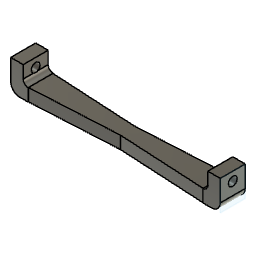
refuerzo estructura brazo elevador (Autodesk Fusion 360 design; units mm, degrees)
Autodesk Fusion 360 part; units mm, degrees
sketch "Sketch1" plane through (0, 0, 0) normal (0, 0, 1) x (1, 0, 0)
  line L0 (0, 0) -> (84, 0)
  line L1 (84, 0) -> (84, 10)
  line L2 (84, 10) -> (0, 10)
  line L3 (0, 10) -> (0, 0)
  dimension "d1" = 84
  dimension "d2" = 10
  constraint horizontal L0
  constraint vertical L1
  constraint horizontal L2
  constraint vertical L3
  constraint coincident L0.start L3.end
  measures "d1" distance of L0.start L0.end
  measures "d2" distance of L0.start L2.end
extrude "Extrude1" add sketch "Sketch1" along normal blind 12
sketch "Sketch2" plane through (0, 0, 0) normal (0, -1, 0) x (1, 0, 0)
  line L0 (0, 0) -> (84, 0)
  line L1 (84, 0) -> (84, 12)
  line L2 (84, 12) -> (0, 12)
  line L3 (0, 12) -> (0, 0)
sketch "Sketch3" plane through (0, 0, 0) normal (0, -1, 0) x (1, 0, 0)
  line L0 (0, 12) -> (5, 12)
  line L1 (5, 12) -> (5, 5)
  line L2 (5, 5) -> (79, 5)
  line L3 (5, 12) -> (6.9617, 12)
  line L4 (6.9617, 12) -> (80, 12)
  line L5 (84, 12) -> (79, 12)
  line L6 (79, 12) -> (79, 5)
  dimension "d5" = 5
  constraint horizontal L0
  constraint perpendicular L0 L1
  constraint perpendicular L1 L2
  constraint perpendicular L1 L3
  constraint parallel L4 L5
  constraint coincident L2 L6.end
  constraint perpendicular L2 L6
  measures "d5" distance of L5.start L5.end
extrude "Extrude2" cut sketch "Sketch3" against normal blind 50
sketch "Sketch4" plane through (84, 0, 0) normal (1, 0, 0) x (0, 1, 0)
  line L0 (0, 0) -> (10, 0)
  line L1 (10, 0) -> (10, 12)
  line L2 (10, 12) -> (0, 12)
  line L3 (0, 12) -> (0, 0)
sketch "Sketch5" plane through (79, 0, 0) normal (-1, 0, 0) x (0, -1, 0)
  line L0 (-10, 12) -> (-10, 5)
  line L1 (-10, 5) -> (0, 5)
  line L2 (0, 5) -> (0, 12)
  line L3 (0, 12) -> (-10, 12)
  circle A0 centre (-5, 8.5) radius 1.75
  dimension "d8" = 3.5
  measures "d8" diameter of A0
extrude "Extrude3" cut sketch "Sketch5" along normal blind 162 and the other way blind 9 contours A0
fillet "Fillet1" radius 3.5 2 edges at (84, 5, 0) (0, 5, 0)
fillet "Fillet2" radius 2 2 edges at (5, 5, 5) (79, 5, 5)
sketch "Sketch6" plane through (0, 0, 5) normal (0, 0, 1) x (-1, 0, 0)
  line L0 (-77, 0) -> (-77, -10)
  line L1 (-77, -10) -> (-7, -10)
  line L2 (-7, -10) -> (-7, 0)
  line L3 (-7, 0) -> (-77, 0)
  line L4 (-42, 0) -> (-42, -2)
  line L5 (-42, -10) -> (-42, -8)
  line L6 (-42, -8) -> (-79, -10)
  line L7 (-42, -2) -> (-79, 0)
  line L8 (-5, 0) -> (-42, -2)
  line L9 (-42, -8) -> (-41, -8)
  line L10 (-41, -8) -> (-5, -10)
  dimension "d17" = 2
  constraint midpoint L3 L4.start
  constraint perpendicular L3 L4
  constraint midpoint L1 L5.start
  constraint perpendicular L1 L5
  constraint perpendicular L5 L9
  measures "d17" distance of L4.start L4.end
extrude "Extrude4" cut sketch "Sketch6" against normal blind 12 contours L0 L3 L4 L7 | L2 L3 L4 L8 | L0 L1 L5 L6 | L1 L2 L5 L9 L10
sketch "Sketch7" plane through (0, 0, 0) normal (0, 1, 0) x (1, 0, 0)
